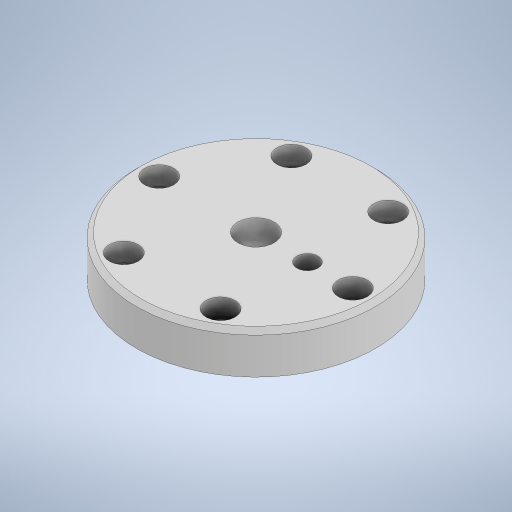
# Autodesk Inventor part: 2_VálvulaSuperior
Saved by Autodesk Inventor 2024.3 (Build 283343000, 343)
## iProperties
Created: 2024-04-26
Part Number: 2_VálvulaSuperior
Material: Genérico
Document SubType Name: Modeling
Designer: Cosmic Dinodog
Density: 1 g/cm^3
Appearance: Valor por defecto
Author: Cosmic Dinodog
Autodesk Inventor part; units mm, degrees
ref_plane "YZ Plane" through (0, 0, 0) normal (1, 0, 0) x (0, 1, 0)
ref_plane "XZ Plane" through (0, 0, 0) normal (0, 1, 0) x (-1, 0, 0)
ref_plane "XY Plane" through (0, 0, 0) normal (0, 0, 1) x (1, 0, 0)
sketch "Boceto1" plane through (0, 0, 0) normal (0, 1, 0) x (-1, 0, 0)
  circle A0 centre (0, 0) radius 79
  circle A1 centre (0, 0) radius 12
  dimension "d0" = 158
  dimension "d1" = 24
  constraints: 2 centre point, 2 coincident
  measures "d0" diameter of A0
  measures "d1" diameter of A1
extrude "Extrusión1" add sketch "Boceto1" along normal blind 27
chamfer "Chaflán1" distance 3 angle 45 1 edges at (79, 27, 0) measured on face at (-12.739, 27, -55.0245)
sketch "Boceto2" plane through (0, 27, 0) normal (0, 1, 0) x (1, 0, 0)
  circle A0 centre (0, 0) radius 64 construction
  line L0 (0, 0) -> (64, 0) construction
  point P0 (32, 55.4256)
  point P1 (-32, 55.4256)
  point P2 (-64, 0)
  point P3 (-32, -55.4256)
  point P4 (32, -55.4256)
  dimension "d7" = 128
  dimension "d10" = 360
  constraints: 2 coincident, 2 end point, 1 horizontal, 1 horizontal alignment, 9 other
hole "Agujero1" at (64, 27, 0) at (32, 27, -55.4256) at (-32, 27, -55.4256) at (-64, 27, 0) at (-32, 27, 55.4256) at (32, 27, 55.4256) direction (0, -1, 0) diameter 12.5 end through all counterbore diameter 19.25 counterbore depth 12.5
sketch "Boceto3" plane through (0, 27, 0) normal (0, 1, 0) x (1, 0, 0)
  line L0 (0, 0) -> (34, 0) construction
  dimension "d19" = 34
  constraints: 2 end point, 1 coincident, 1 horizontal
  measures "d19" distance of L0.start L0.end
hole "Agujero2" at (34, 27, 0) direction (0, -1, 0) diameter 14 depth 17
sketch "Boceto5" plane through (0, 0, 0) normal (0, 0, 1) x (1, 0, 0)
  line L0 (79, 0) -> (-79, 0) construction
  line L1 (79, 0) -> (33, 0) construction
  line L2 (33, 0) -> (44, 0)
  line L3 (44, 0) -> (44, 6)
  line L4 (44, 6) -> (33, 6)
  line L5 (33, 6) -> (33, 0)
  line L6 (0, 0) -> (0, 42.6021) construction
  dimension "d29" = 46
  dimension "d30" = 11
  dimension "d31" = 6
  dimension "d32" = 11
  constraints: 12 end point, 2 perpendicular, 2 point on line, 1 vertical
  measures "d29" distance of L0.start L1.end
  measures "d30" distance of L1.end L2.end
  measures "d31" distance of L2.end L3.end
  measures "d32" distance of L3.end L4.end
revolve "Revolución1" cut sketch "Boceto5" angle 360 about axis through (0, 0, 0) along (0, 1, 0)
